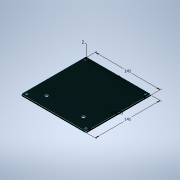
# Autodesk Inventor part: plate_f16
Saved by Autodesk Inventor 2021 (Build 250183000, 183)
## iProperties
Created: 2023-12-15
Part Number: plate_f16
Material: Generic
Document SubType Name: Modeling
Designer: assman
Density: 1 g/cm^3
Appearance: Aluminum - Flat
Author: assman
Autodesk Inventor part; units mm, degrees
ref_plane "YZ Plane" through (0, 0, 0) normal (1, 0, 0) x (0, 1, 0)
ref_plane "XZ Plane" through (0, 0, 0) normal (0, 1, 0) x (-1, 0, 0)
ref_plane "XY Plane" through (0, 0, 0) normal (0, 0, 1) x (1, 0, 0)
sketch "Sketch1" plane through (0, 0, 0) normal (0, 1, 0) x (-1, 0, 0)
  line L0 (64.5, 64.625) -> (-64.5, 64.625) construction
  line L1 (-64.5, 64.625) -> (-64.5, -64.625) construction
  line L2 (-64.5, -64.625) -> (62.5, -64.625) construction
  line L3 (64.5, -62.625) -> (64.5, 64.625) construction
  line L4 (64.5, 64.625) -> (-64.5, -64.625) construction
  line L5 (-64.5, 64.625) -> (64.5, -64.625) construction
  line L6 (68.5, 70.5) -> (-68.5, 70.5)
  line L7 (-70.5, 68.5) -> (-70.5, -68.5)
  line L8 (-68.5, -70.5) -> (68.5, -70.5)
  line L9 (70.5, -68.5) -> (70.5, 68.5)
  line L10 (70.5, 70.5) -> (-70.5, -70.5) construction
  line L11 (-70.5, 70.5) -> (70.5, -70.5) construction
  arc A0 (62.5, -64.625) -> (64.5, -62.625) centre (62.5, -62.625) ccw
  arc A1 (70.5, 68.5) -> (68.5, 70.5) centre (68.5, 68.5) ccw
  arc A2 (68.5, -70.5) -> (70.5, -68.5) centre (68.5, -68.5) ccw
  arc A3 (-70.5, -68.5) -> (-68.5, -70.5) centre (-68.5, -68.5) ccw
  arc A4 (-68.5, 70.5) -> (-70.5, 68.5) centre (-68.5, 68.5) ccw
  point P0 (0, 0)
  dimension "d0" = 129
  dimension "d1" = 129.25
  dimension "d2" = 141
  dimension "d3" = 141
  dimension "d4" = 2
  constraints: 24 end point, 10 point on circle, 10 point on line, 10 tangent, 5 centre point, 4 coincident, 4 equal radius, 4 midpoint, 4 parallel, 2 horizontal, 2 perpendicular
  measures "d0" distance of L5.end L1.end
  measures "d1" distance of L1.end L0.end
  measures "d2" distance of L11.end L10.end
  measures "d3" distance of L10.end L11.start
  measures "d4" radius of A0
extrude "Extrusion1" add sketch "Sketch1" along normal blind 2
hole "Hole1" at (64.5, 0, -64.625) at (64.5, 0, 64.625) at (-64.5, 0, -64.625) at (-64.5, 0, 64.625) direction (0, 1, 0) diameter 4 end through all
sketch "Sketch2" plane through (0, 2, 0) normal (0, 1, 0) x (1, 0, 0)
  circle A0 centre (-64.5, 64.625) radius 2 construction
  circle A1 centre (64.5, 64.625) radius 2 construction
  circle A2 centre (64.5, -64.625) radius 2 construction
  circle A3 centre (-64.5, -64.625) radius 2 construction
  arc A4 (68.5, -70.5) -> (70.5, -68.5) centre (68.5, -68.5) ccw construction
  line L0 (70.5, -68.5) -> (70.5, 68.5) construction
  arc A5 (70.5, 68.5) -> (68.5, 70.5) centre (68.5, 68.5) ccw construction
  line L1 (68.5, 70.5) -> (-68.5, 70.5) construction
  arc A6 (-68.5, 70.5) -> (-70.5, 68.5) centre (-68.5, 68.5) ccw construction
  line L2 (-70.5, 68.5) -> (-70.5, -68.5) construction
  arc A7 (-70.5, -68.5) -> (-68.5, -70.5) centre (-68.5, -68.5) ccw construction
  line L3 (-68.5, -70.5) -> (68.5, -70.5) construction
  line L4 (70.5, -68.5) -> (70.5, 68.5) construction
  line L5 (70.5, -45.5) -> (-70.5, -45.5) construction
  line L6 (-70.5, 68.5) -> (-70.5, -68.5) construction
  line L7 (0, -45.5) -> (-40, -45.5) construction
  line L8 (-40, -45.5) -> (0, -45.5) construction
  line L9 (0, -45.5) -> (40, -45.5) construction
  point P0 (0, 0)
  dimension "d14" = 25
  dimension "d15" = 40
  dimension "d16" = 40
  constraints: 8 end point, 4 point on line, 2 coincident, 1 collinear, 1 midpoint, 1 perpendicular
  measures "d14" distance between parallel lines of L3 L5
  measures "d15" distance of L7.start L7.end
  measures "d16" distance of L7.start L9.end
hole "Hole2" at (-40, 2, 45.5) at (40, 2, 45.5) direction (0, -1, 0) diameter 4 end through all countersink diameter 6 countersink angle 90
body "Solid1"
